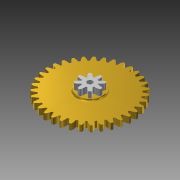
# Autodesk Inventor part: 2ndreductor
Saved by Autodesk Inventor 2014 SP1 (Build 180222100, 222)
## iProperties
Created: 2017-09-24
Part Number: 2ndreductor
Material: Steel
Document SubType Name: Modeling
Designer: Vivi
Categories: <?xml version="1.0" encoding="UTF-16"?> <MemberInstance><Categories><FamilyTemplate><FamilyTemplateParameter ValueType="xs:double" Id="1" ObjectReferenceKey="da_z" ObjectType="kUserParameterObject"/><FamilyTemplateParameter ValueType="xs:double" Id="2" ObjectReferenceKey="da_b" ObjectType="kUserParameterObject"/><FamilyTemplateParameter ValueType="xs:double" Id="3" ObjectReferenceKey="da_beta" ObjectType="kUserParameterObject"/><FamilyTemplateParameter ValueType="xs:double" Id="4" ObjectReferenceKey="da_da" ObjectType="kUserParameterObject"/><FamilyTemplateParameter ValueType="xs:double" Id="5" ObjectReferenceKey="da_aw" ObjectType="kUserParameterObject"/><FamilyTemplateParameter ValueType="xs:string" Id="6" ObjectReferenceKey="EAIAABAAAACIAQAAAAAAAIAAAAAAAAAA" ObjectType="83910656" SubObjectId="SurfaceGeometry"/></FamilyTemplate><ParamToTemplateMap><ParamToTemplate CategoryParameter="//CategoryParameter[@InternalName='046C89C9-8512-4d59-83FE-43B91F4F132A']" TemplateParameter="1"/><ParamToTemplate CategoryParameter="//CategoryParameter[@InternalName='2552DF32-E462-4b46-AEBF-C6C7768E72AC']" TemplateParameter="2"/><ParamToTemplate CategoryParameter="//CategoryParameter[@InternalName='C9EE641D-15FC-4fae-A226-E94C4372FDD7']" TemplateParameter="3"/><ParamToTemplate><ParamToTemplate CategoryParameter="//CategoryParameter[@InternalName='00B6519A-459B-49c7-AD84-2E56D39A5744']" ConstantValue="0.000000"/></ParamToTemplate><ParamToTemplate><ParamToTemplate CategoryParameter="//CategoryParameter[@InternalName='04B31F0E-C7A6-4894-AA32-9629BEFACF47']" ConstantValue="1.000000"/></ParamToTemplate><ParamToTemplate><ParamToTemplate CategoryParameter="//CategoryParameter[@InternalName='43CBEC2E-7847-49e7-A936-2F7889FCB2D9']" ConstantValue="0.250000"/></ParamToTemplate><ParamToTemplate><ParamToTemplate CategoryParameter="//CategoryParameter[@InternalName='B1EFC894-105D-4ebd-86BF-FA20ED196853']" ConstantValue="0.350000"/></ParamToTemplate><ParamToTemplate><ParamToTemplate CategoryParameter="//CategoryParameter[@InternalName='51175063-3D10-4879-93E8-6246FE8B403D']" ConstantValue="2060000000.000000"/></ParamToTemplate><ParamToTemplate><ParamToTemplate CategoryParameter="//CategoryParameter[@InternalName='A3A52E27-4454-46a9-B0BD-C932399B70AF']" ConstantValue="0.300000"/></ParamToTemplate><ParamToTemplate><ParamToTemplate CategoryParameter="//CategoryParameter[@InternalName='91B76062-C214-41d9-B1B9-14D2AB99603D']" ConstantValue="0.150000"/></ParamToTemplate><ParamToTemplate><ParamToTemplate CategoryParameter="//CategoryParameter[@InternalName='374E806E-8B8A-4dda-A9AA-1039D6500AD2']" ConstantValue="6.666667"/></ParamToTemplate><ParamToTemplate><ParamToTemplate CategoryParameter="//CategoryParameter[@InternalName='2D373A89-B862-43d6-8D0B-0CBF12AB9F6C']" ConstantValue="0.523599"/></ParamToTemplate><ParamToTemplate CategoryParameter="//CategoryParameter[@InternalName='37777632-D6A2-4fac-9D53-DB8ACD95C989']" TemplateParameter="4"/><ParamToTemplate CategoryParameter="//CategoryParameter[@InternalName='FD1017F1-B727-4f7e-9707-0F86F1FF9423']" TemplateParameter="5"/><ParamToTemplate><ParamToTemplate CategoryParameter="//CategoryParameter[@InternalName='9E1B4470-B2D3-4ff1-B813-535BB4CDF51A']" ConstantValue="3520000.000000"/></ParamToTemplate><ParamToTemplate><ParamToTemplate CategoryParameter="//CategoryParameter[@InternalName='F8452263-BFF6-458c-9FB1-07C4B99E95CD']" ConstantValue="11400000.000000"/></ParamToTemplate><ParamToTemplate><ParamToTemplate CategoryParameter="//CategoryParameter[@InternalName='3E3BB259-FD49-497f-8171-6EBC954A3479']" ConstantValue="2.000000"/></ParamToTemplate><ParamToTemplate CategoryParameter="//CategoryParameter[@InternalName='27C3BAF2-7550-4e4b-AE2C-0DB134B7D9B7']" TemplateParameter="6"/></ParamToTemplateMap><Category DisplayName="Gear" InternalName="DC85795E-93AB-48d5-8EEE-5A27447B64BD" Mnemonic="Gear"><CategoryParameter DisplayName="z" InternalName="046C89C9-8512-4d59-83FE-43B91F4F132A" Mnemonic="z"/><CategoryParameter DisplayName="b" InternalName="2552DF32-E462-4b46-AEBF-C6C7768E72AC" Mnemonic="b"/><CategoryParameter DisplayName="||b|" InternalName="C9EE641D-15FC-4fae-A226-E94C4372FDD7" Mnemonic="beta"/><CategoryParameter DisplayName="x" InternalName="00B6519A-459B-49c7-AD84-2E56D39A5744" Mnemonic="x"/><CategoryParameter DisplayName="a*" InternalName="04B31F0E-C7A6-4894-AA32-9629BEFACF47" Mnemonic="a"/><CategoryParameter DisplayName="c*" InternalName="43CBEC2E-7847-49e7-A936-2F7889FCB2D9" Mnemonic="c"/><CategoryParameter DisplayName="r|.f|*" InternalName="B1EFC894-105D-4ebd-86BF-FA20ED196853" Mnemonic="rf"/><CategoryParameter DisplayName="E" InternalName="51175063-3D10-4879-93E8-6246FE8B403D" Mnemonic="E"/><CategoryParameter DisplayName="||m|" InternalName="A3A52E27-4454-46a9-B0BD-C932399B70AF" Mnemonic="mi"/><Category DisplayName="SpurGear" InternalName="26C5A22E-A91E-4dfd-A3B3-23CCAFAE1764" Mnemonic="SpurGear"><CategoryParameter DisplayName="m" InternalName="91B76062-C214-41d9-B1B9-14D2AB99603D" Mnemonic="m"/><CategoryParameter DisplayName="P" InternalName="374E806E-8B8A-4dda-A9AA-1039D6500AD2" Mnemonic="PP"/><CategoryParameter DisplayName="||a|" InternalName="2D373A89-B862-43d6-8D0B-0CBF12AB9F6C" Mnemonic="alpha"/><CategoryParameter DisplayName="d|.a|" InternalName="37777632-D6A2-4fac-9D53-DB8ACD95C989" Mnemonic="da"/><CategoryParameter DisplayName="a|.w|" InternalName="FD1017F1-B727-4f7e-9707-0F86F1FF9423" Mnemonic="aw"/><CategoryParameter DisplayName="||s||.Flim|" InternalName="9E1B4470-B2D3-4ff1-B813-535BB4CDF51A" Mnemonic="sFlim"/><CategoryParameter DisplayName="||s||.Hlim|" InternalName="F8452263-BFF6-458c-9FB1-07C4B99E95CD" Mnemonic="sHlim"/><CategoryParameter DisplayName="type" InternalName="3E3BB259-FD49-497f-8171-6EBC954A3479" Mnemonic="type"/><CategoryParameter DisplayName="PitchDiameter" InternalName="27C3BAF2-7550-4e4b-AE2C-0DB134B7D9B7" Mnemonic="IDS_PITCHDIAM"/></Category></Category></Categories></MemberInstance>
Density: 1 g/cm^3
Appearance: Steel
CustomPartVersion: 1
Author: Vivi
Autodesk Inventor part; units mm, degrees
sketch "Sketch1" plane through (0, 0, 0) normal (0, 0, 1) x (1, 0, 0)
  circle A0 centre (0, 0) radius 27.75
  dimension "d0" = 55.5
  constraints: 1 centre point
  measures "d0" diameter of A0
extrude "Extrusion1" add sketch "Sketch1" along normal blind 4
ref_plane "Work Plane2" through (0, 0, 2) normal (0, 0, 1) x (1, 0, 0)
sketch "Sketch2" plane through (0, 0, 0) normal (0, 0, -1) x (-1, 0, 0)
  circle A0 centre (0, 0) radius 27.75 projected
  circle A1 centre (0, 0) radius 26.25
  dimension "d3" = 52.5
  constraints: 1 centre point, 1 coincident
  measures "d3" diameter of A1
surface extrude "Pitch Diameter" sketch "Sketch2" against normal through all shown no curves A1
ref_plane "Work Plane8" through (0, 0, 0) normal (0.9959743, 0.0896393, 0) x (0, 0, 1)
ref_plane "Work Plane9" through (0, 0, 0) normal (1, 0, 0) x (0, 1, 0)
spur gear teeth "Spur Gear" teeth 35 pitch diameter 52.5 tip diameter 55.5 root diameter 48.75 face width 10 start plane through (0, 0, 0) normal (0, 0, -1) x (-1, 0, 0)
sketch "Sketch3" plane through (0, 0, 4) normal (0, 0, 1) x (1, 0, 0)
  circle A0 centre (0, 0) radius 1.1
  arc A1 (3.6379, 1.9445) -> (5.7976, 4.7579) centre (-0.6751, 7.4909) ccw
  arc A2 (5.7976, 4.7579) -> (4.7579, 5.7976) centre (0, 0) ccw
  arc A3 (4.7579, 5.7976) -> (1.9445, 3.6379) centre (7.4909, -0.6751) ccw
  arc A4 (1.9445, 3.6379) -> (1.1974, 3.9474) centre (0, 0) ccw
  arc A5 (1.1974, 3.9474) -> (0.7351, 7.4639) centre (-5.7742, 4.8195) ccw
  arc A6 (0.7351, 7.4639) -> (-0.7351, 7.4639) centre (0, 0) ccw
  arc A7 (-0.7351, 7.4639) -> (-1.1974, 3.9474) centre (5.7742, 4.8195) ccw
  arc A8 (-1.1974, 3.9474) -> (-1.9445, 3.6379) centre (0, 0) ccw
  arc A9 (-1.9445, 3.6379) -> (-4.7579, 5.7976) centre (-7.4909, -0.6751) ccw
  arc A10 (-4.7579, 5.7976) -> (-5.7976, 4.7579) centre (0, 0) ccw
  arc A11 (-5.7976, 4.7579) -> (-3.6379, 1.9445) centre (0.6751, 7.4909) ccw
  arc A12 (-3.6379, 1.9445) -> (-3.9474, 1.1974) centre (0, 0) ccw
  arc A13 (-3.9474, 1.1974) -> (-7.4639, 0.7351) centre (-4.8195, -5.7742) ccw
  arc A14 (-7.4639, 0.7351) -> (-7.4639, -0.7351) centre (0, 0) ccw
  arc A15 (-7.4639, -0.7351) -> (-3.9474, -1.1974) centre (-4.8195, 5.7742) ccw
  arc A16 (-3.9474, -1.1974) -> (-3.6379, -1.9445) centre (0, 0) ccw
  arc A17 (-3.6379, -1.9445) -> (-5.7976, -4.7579) centre (0.6751, -7.4909) ccw
  arc A18 (-5.7976, -4.7579) -> (-4.7579, -5.7976) centre (0, 0) ccw
  arc A19 (-4.7579, -5.7976) -> (-1.9445, -3.6379) centre (-7.4909, 0.6751) ccw
  arc A20 (-1.9445, -3.6379) -> (-1.1974, -3.9474) centre (0, 0) ccw
  arc A21 (-1.1974, -3.9474) -> (-0.7351, -7.4639) centre (5.7742, -4.8195) ccw
  arc A22 (-0.7351, -7.4639) -> (0.7351, -7.4639) centre (0, 0) ccw
  arc A23 (0.7351, -7.4639) -> (1.1974, -3.9474) centre (-5.7742, -4.8195) ccw
  arc A24 (1.1974, -3.9474) -> (1.9445, -3.6379) centre (0, 0) ccw
  arc A25 (1.9445, -3.6379) -> (4.7579, -5.7976) centre (7.4909, 0.6751) ccw
  arc A26 (4.7579, -5.7976) -> (5.7976, -4.7579) centre (0, 0) ccw
  arc A27 (5.7976, -4.7579) -> (3.6379, -1.9445) centre (-0.6751, -7.4909) ccw
  arc A28 (3.6379, -1.9445) -> (3.9474, -1.1974) centre (0, 0) ccw
  arc A29 (3.9474, -1.1974) -> (7.4639, -0.7351) centre (4.8195, 5.7742) ccw
  arc A30 (7.4639, -0.7351) -> (7.4639, 0.7351) centre (0, 0) ccw
  arc A31 (7.4639, 0.7351) -> (3.9474, 1.1974) centre (4.8195, -5.7742) ccw
  arc A32 (3.9474, 1.1974) -> (3.6379, 1.9445) centre (0, 0) ccw
  circle A33 centre (0, 0) radius 1.75
  dimension "d49" = 3.5
  constraints: 64 point on circle, 34 centre point, 1 coincident
  measures "d49" diameter of A33
extrude "Extrusion2" add sketch "Sketch3" along normal blind 5 contours A32 A31 A30 A29 A28 A27 A26 A25 A24 A23 A22 A21 A20 A19 A18 A17 A16 A15 A14 A13 A12 A11 A10 A9 A8 A7 A6 A5 A4 A3 A2 A1
sketch "Sketch4" plane through (0, 0, 4) normal (0, 0, 1) x (1, 0, 0)
  circle A0 centre (0, 0) radius 1.75 projected
extrude "Extrusion3" cut sketch "Sketch4" against normal blind 10
sketch "Sketch6" plane through (0, 0, 4) normal (0, 0, 1) x (1, 0, 0)
  arc A0 (0.7351, 7.4639) -> (-0.7351, 7.4639) centre (0, 0) ccw projected
  arc A1 (1.1974, 3.9474) -> (0.7351, 7.4639) centre (-5.7742, 4.8195) ccw projected
  arc A2 (1.9445, 3.6379) -> (1.1974, 3.9474) centre (0, 0) ccw projected
  arc A3 (4.7579, 5.7976) -> (1.9445, 3.6379) centre (7.4909, -0.6751) ccw projected
  arc A4 (5.7976, 4.7579) -> (4.7579, 5.7976) centre (0, 0) ccw projected
  arc A5 (3.6379, 1.9445) -> (5.7976, 4.7579) centre (-0.6751, 7.4909) ccw projected
  arc A6 (3.9474, 1.1974) -> (3.6379, 1.9445) centre (0, 0) ccw projected
  arc A7 (7.4639, 0.7351) -> (3.9474, 1.1974) centre (4.8195, -5.7742) ccw projected
  arc A8 (7.4639, -0.7351) -> (7.4639, 0.7351) centre (0, 0) ccw projected
  arc A9 (3.9474, -1.1974) -> (7.4639, -0.7351) centre (4.8195, 5.7742) ccw projected
  arc A10 (3.6379, -1.9445) -> (3.9474, -1.1974) centre (0, 0) ccw projected
  arc A11 (5.7976, -4.7579) -> (3.6379, -1.9445) centre (-0.6751, -7.4909) ccw projected
  arc A12 (4.7579, -5.7976) -> (5.7976, -4.7579) centre (0, 0) ccw projected
  arc A13 (1.9445, -3.6379) -> (4.7579, -5.7976) centre (7.4909, 0.6751) ccw projected
  arc A14 (1.1974, -3.9474) -> (1.9445, -3.6379) centre (0, 0) ccw projected
  arc A15 (0.7351, -7.4639) -> (1.1974, -3.9474) centre (-5.7742, -4.8195) ccw projected
  arc A16 (-0.7351, -7.4639) -> (0.7351, -7.4639) centre (0, 0) ccw projected
  arc A17 (-1.1974, -3.9474) -> (-0.7351, -7.4639) centre (5.7742, -4.8195) ccw projected
  arc A18 (-1.9445, -3.6379) -> (-1.1974, -3.9474) centre (0, 0) ccw projected
  arc A19 (-4.7579, -5.7976) -> (-1.9445, -3.6379) centre (-7.4909, 0.6751) ccw projected
  arc A20 (-5.7976, -4.7579) -> (-4.7579, -5.7976) centre (0, 0) ccw projected
  arc A21 (-3.6379, -1.9445) -> (-5.7976, -4.7579) centre (0.6751, -7.4909) ccw projected
  arc A22 (-3.9474, -1.1974) -> (-3.6379, -1.9445) centre (0, 0) ccw projected
  arc A23 (-7.4639, -0.7351) -> (-3.9474, -1.1974) centre (-4.8195, 5.7742) ccw projected
  arc A24 (-7.4639, 0.7351) -> (-7.4639, -0.7351) centre (0, 0) ccw projected
  arc A25 (-3.9474, 1.1974) -> (-7.4639, 0.7351) centre (-4.8195, -5.7742) ccw projected
  arc A26 (-3.6379, 1.9445) -> (-3.9474, 1.1974) centre (0, 0) ccw projected
  arc A27 (-5.7976, 4.7579) -> (-3.6379, 1.9445) centre (0.6751, 7.4909) ccw projected
  arc A28 (-4.7579, 5.7976) -> (-5.7976, 4.7579) centre (0, 0) ccw projected
  arc A29 (-1.9445, 3.6379) -> (-4.7579, 5.7976) centre (-7.4909, -0.6751) ccw projected
  arc A30 (-1.1974, 3.9474) -> (-1.9445, 3.6379) centre (0, 0) ccw projected
  arc A31 (-0.7351, 7.4639) -> (-1.1974, 3.9474) centre (5.7742, 4.8195) ccw projected
  circle A32 centre (0, 0) radius 8
  dimension "d54" = 16
  constraints: 1 centre point, 1 coincident
  measures "d54" diameter of A32
extrude "Extrusion4" add sketch "Sketch6" along normal blind 1
fillet "Fillet1" radius 1 1 edges at (-8, 0, 4)
equation "\"d0\" = da_da"
equation "\"d3\" = da_dw"
equation "\"d16\" = da_aw"
equation "\"d43\" = da_aw"
equation "\"d46\" = da_aw"
equation "\"da_da\" = 55.5"
equation "\"da_dw\" = 52.5"
equation "\"da_aw\" = 222.75"
body "Solid1"
body "Srf1"
